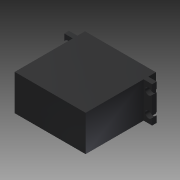
# Autodesk Inventor part: servo 33kg TGY-S8166M
Saved by Autodesk Inventor 2013 (Build 170138000, 138)
## iProperties
Created: 2013-03-06
Part Number: servo 33kg TGY-S8166M
Material: Generic
Document SubType Name: Modeling
Designer: Masta
Density: 1.41898 g/cm^3
Mass: 160 g
Surface Area: 160.569 cm^2
Volume: 112.757 cm^3
Author: Masta
Autodesk Inventor part; units mm, degrees
ref_plane "YZ Plane" through (0, 0, 0) normal (1, 0, 0) x (0, 1, 0)
ref_plane "XZ Plane" through (0, 0, 0) normal (0, 1, 0) x (-1, 0, 0)
ref_plane "XY Plane" through (0, 0, 0) normal (0, 0, 1) x (1, 0, 0)
sketch "Sketch1" plane through (0, 0, 0) normal (0, 1, 0) x (-1, 0, 0)
  line L0 (30.25, 15.25) -> (-30.25, 15.25)
  line L1 (-30.25, 15.25) -> (-30.25, -15.25)
  line L2 (-30.25, -15.25) -> (30.25, -15.25)
  line L3 (30.25, -15.25) -> (30.25, 15.25)
  line L4 (30.25, 15.25) -> (-30.25, -15.25) construction
  line L5 (-30.25, 15.25) -> (30.25, -15.25) construction
  line L6 (-37.5, 15.25) -> (-37.5, 9.75)
  line L7 (37.5, -15.25) -> (37.5, -9.75)
  line L8 (37.5, 15.25) -> (-37.5, -15.25) construction
  line L9 (-37.5, 15.25) -> (37.5, -15.25) construction
  line L10 (30.25, -15.25) -> (37.5, -15.25)
  line L11 (30.25, 15.25) -> (37.5, 15.25)
  line L12 (-30.25, 15.25) -> (-37.5, 15.25)
  line L13 (-30.25, -15.25) -> (-37.5, -15.25)
  line L14 (34.5, 8.5) -> (-34.5, 8.5) construction
  line L15 (-34.5, 8.5) -> (-34.5, -8.5) construction
  line L16 (-34.5, -8.5) -> (34.5, -8.5) construction
  line L17 (34.5, -8.5) -> (34.5, 8.5) construction
  line L18 (34.5, 8.5) -> (-34.5, -8.5) construction
  line L19 (-34.5, 8.5) -> (34.5, -8.5) construction
  circle A0 centre (-34.5, 8.5) radius 3
  line L20 (-37.5, 7.25) -> (-37.2272, 7.25)
  line L21 (-37.5, 9.75) -> (-37.2272, 9.75)
  line L22 (-30.25, 0) -> (30.25, 0) construction
  line L23 (0, 15.25) -> (0, -15.25) construction
  circle A1 centre (-34.5, -8.5) radius 3
  line L24 (-37.5, -7.25) -> (-37.2272, -7.25)
  line L25 (-37.5, -9.75) -> (-37.2272, -9.75)
  circle A2 centre (34.5, 8.5) radius 3
  line L26 (37.5, 7.25) -> (37.2272, 7.25)
  line L27 (37.5, 9.75) -> (37.2272, 9.75)
  line L28 (37.5, -9.75) -> (37.2272, -9.75)
  line L29 (37.5, -7.25) -> (37.2272, -7.25)
  circle A3 centre (34.5, -8.5) radius 3
  line L30 (-37.5, 7.25) -> (-37.5, -7.25)
  line L31 (-37.5, 9.75) -> (-37.5, 7.25)
  line L32 (-37.5, -9.75) -> (-37.5, -15.25)
  line L33 (-37.5, -7.25) -> (-37.5, -9.75)
  line L34 (37.5, -7.25) -> (37.5, 7.25)
  line L35 (37.5, -9.75) -> (37.5, -7.25)
  line L36 (37.5, 7.25) -> (37.5, 9.75)
  line L37 (37.5, 9.75) -> (37.5, 15.25)
  point P0 (0, 0)
  dimension "d0" = 60.5
  dimension "d1" = 30.5
  dimension "d2" = 75
  dimension "d3" = 69
  dimension "d4" = 17
  dimension "d12" = 2.5
  dimension "d13" = 6
  constraints: 76 end point, 32 parallel, 15 symmetric about line, 12 perpendicular, 10 midpoint, 8 point on circle, 4 centre point, 2 collinear, 2 horizontal, 1 coincident, 4 other
  measures "d0" distance of L2.end L1.end
  measures "d1" distance of L1.end L0.end
  measures "d2" distance of L7.start L8.end
  measures "d3" distance of L16.end L15.end
  measures "d4" distance of L15.end L14.end
  measures "d12" distance between parallel lines of L20 L21
  measures "d13" diameter of A0
extrude "Extrusion1" add sketch "Sketch1" along normal blind 10.5 and the other way blind 49.5 contours L3 L2 L1 L0
extrude "Extrusion2" add sketch "Sketch1" along normal blind 4 contours L11 L37 L27 A2 L26 L34 L29 A3 L28 L7 L10 L3 | L1 L13 L32 L25 A1 L24 L30 L20 A0 L21 L6 L12
sketch "Sketch2" plane through (0, 10.5, 0) normal (0, 1, 0) x (1, 0, 0)
  line L0 (-30.25, 15.25) -> (-30.25, -15.25) projected
  circle A0 centre (-15.25, 0) radius 7.5
  line L1 (-15.25, 0) -> (0, 0) construction
  dimension "d14" = 15
  dimension "d15" = 15
  constraints: 2 end point, 1 centre point, 1 perpendicular
  measures "d14" diameter of A0
  measures "d15" distance from line of L1.start L0
extrude "Extrusion3" add sketch "Sketch2" along normal blind 2
sketch "Sketch3" plane through (-15.25, 12.5, 0) normal (0, 1, 0) x (1, 0, 0)
  circle A0 centre (0, 0) radius 7.5 projected
  circle A1 centre (0, 0) radius 3.5
  point P0 (15.25, 0)
  dimension "d18" = 7
  constraints: 1 centre point, 1 coincident
  measures "d18" diameter of A1
extrude "Extrusion4" add sketch "Sketch3" along normal blind 6 contours A1
sketch "Sketch4" plane through (-30.25, -49.5, -15.25) normal (-1, 0, 0) x (0, 0, 1)
  line L0 (30.5, 49.5) -> (0, 49.5) projected
  line L1 (11.75, 25) -> (18.75, 25)
  line L2 (18.75, 25) -> (18.75, 29.5)
  line L3 (18.75, 29.5) -> (11.75, 29.5)
  line L4 (11.75, 29.5) -> (11.75, 25)
  line L5 (11.75, 25) -> (18.75, 29.5) construction
  line L6 (18.75, 25) -> (11.75, 29.5) construction
  line L7 (15.25, 49.5) -> (15.25, 27.25) construction
  dimension "d21" = 7
  dimension "d22" = 4.5
  dimension "d23" = 20
  constraints: 14 end point, 3 parallel, 2 midpoint, 1 horizontal, 1 perpendicular
  measures "d21" distance of L3.end L2.end
  measures "d22" distance of L2.end L1.end
  measures "d23" distance between parallel lines of L0 L3
extrude "Extrusion5" add sketch "Sketch4" along normal blind 7 draft -5
sketch "Sketch5" plane through (0, 0, 0) normal (0, 0, 1) x (1, 0, 0)
  line L0 (37.5, 4) -> (37.5, 0) projected
  line L1 (37.5, 0) -> (30.25, 0) projected
  line L2 (30.25, 0) -> (30.25, -49.5) projected
  line L3 (30.25, -49.5) -> (-30.25, -49.5) projected
  line L4 (-30.25, -24.5) -> (-37.25, -23.8876) projected
  line L5 (-37.25, -23.8876) -> (-37.25, -20.6124) projected
  line L6 (-37.25, -20.6124) -> (-30.25, -20) projected
  line L7 (-30.25, -20) -> (-30.25, 0) projected
  line L8 (-30.25, 0) -> (-37.5, 0) projected
  line L9 (-37.5, 0) -> (-37.5, 4) projected
  line L10 (-37.5, 4) -> (-30.25, 4) projected
  line L11 (-30.25, 4) -> (-30.25, 10.5) projected
  line L12 (-30.25, 10.5) -> (-22.75, 10.5) projected
  line L13 (-22.75, 10.5) -> (-22.75, 12.5) projected
  line L14 (-22.75, 12.5) -> (-18.75, 12.5) projected
  line L15 (-18.75, 12.5) -> (-18.75, 18.5) projected
  line L16 (-18.75, 18.5) -> (-11.75, 18.5) projected
  line L17 (-11.75, 18.5) -> (-11.75, 12.5) projected
  line L18 (-11.75, 12.5) -> (-7.75, 12.5) projected
  line L19 (-7.75, 12.5) -> (-7.75, 10.5) projected
  line L20 (-7.75, 10.5) -> (30.25, 10.5) projected
  line L21 (30.25, 10.5) -> (30.25, 4) projected
  line L22 (30.25, 4) -> (37.5, 4) projected
  line L23 (-37.5, 4) -> (-30.25, 5.1)
  line L24 (30.25, 5.1) -> (37.5, 4)
  line L25 (-30.25, -49.5) -> (-30.25, -24.5) projected
  point P0 (0, 0)
  point P1 (-20.25, -27)
  dimension "d26" = 1.1
  constraints: 4 end point, 2 point on line, 1 equal length
  measures "d26" distance of L23.end L10.end
extrude "Extrusion6" add sketch "Sketch5" along normal mid plane 1.3 contours L22 L21 L24 | L23 L11 L10
sketch "Sketch6" plane through (0, 10.5, 0) normal (0, 1, 0) x (1, 0, 0)
  line L0 (12.3297, -9.4801) -> (12.3297, 4.6475) construction
  line L1 (12.3297, 4.6475) -> (15.9034, 4.6475) construction
  line L2 (15.9034, 4.6475) -> (15.9034, -9.4801) construction
  line L3 (15.9034, -9.4801) -> (12.3297, -9.4801) construction
  line L4 (14.8586, -8.6525) -> (12.6784, -8.6525)
  line L5 (12.6784, -8.6525) -> (12.6784, -9.4821)
  line L6 (12.6784, -9.4821) -> (12.3858, -9.4821)
  line L7 (12.3858, -9.4821) -> (12.3858, -7.4942)
  line L8 (12.3858, -7.4942) -> (12.6784, -7.4942)
  line L9 (12.6784, -7.4942) -> (12.6784, -8.3238)
  line L10 (12.6784, -8.3238) -> (14.8586, -8.3238)
  line L11 (14.8586, -8.3238) -> (14.8586, -8.6525)
  spline S0 degree 2 poles (14.9067, -6.2077) (14.9067, -6.4702) (14.7464, -6.9051) (14.5841, -7.0614) knots 0 0 0 1 2 2 2
  spline S1 degree 2 poles (14.5841, -7.0614) (14.4198, -7.2177) (13.9348, -7.384) (13.6202, -7.384) knots 0 0 0 1 2 2 2
  spline S2 degree 2 poles (13.6202, -7.384) (13.3216, -7.384) (12.8487, -7.2157) (12.6804, -7.0594) knots 0 0 0 1 2 2 2
  spline S3 degree 2 poles (12.6804, -7.0594) (12.5181, -6.9091) (12.3417, -6.4682) (12.3417, -6.2057) knots 0 0 0 1 2 2 2
  spline S4 degree 2 poles (12.3417, -6.2057) (12.3417, -6.0795) (12.3778, -5.851) (12.4098, -5.7468) knots 0 0 0 1 2 2 2
  spline S5 degree 2 poles (12.4098, -5.7468) (12.4339, -5.6627) (12.5221, -5.4583) (12.5541, -5.3961) knots 0 0 0 1 2 2 2
  line L12 (12.5541, -5.3961) -> (12.9509, -5.3961)
  line L13 (12.9509, -5.3961) -> (12.9509, -5.4242)
  spline S6 degree 2 poles (12.9509, -5.4242) (12.8968, -5.4863) (12.7986, -5.6166) (12.7425, -5.7368) knots 0 0 0 1 2 2 2
  spline S7 degree 2 poles (12.7425, -5.7368) (12.6924, -5.837) (12.6263, -6.0955) (12.6263, -6.2438) knots 0 0 0 1 2 2 2
  spline S8 degree 2 poles (12.6263, -6.2438) (12.6263, -6.6005) (13.1633, -7.0413) (13.6102, -7.0413) knots 0 0 0 1 2 2 2
  spline S9 degree 2 poles (13.6102, -7.0413) (13.8587, -7.0413) (14.2314, -6.9251) (14.3596, -6.8149) knots 0 0 0 1 2 2 2
  spline S10 degree 2 poles (14.3596, -6.8149) (14.4879, -6.7087) (14.6222, -6.4081) (14.6222, -6.2197) knots 0 0 0 1 2 2 2
  spline S11 degree 2 poles (14.6222, -6.2197) (14.6222, -6.0815) (14.5821, -5.8049) (14.542, -5.7107) knots 0 0 0 1 2 2 2
  line L14 (14.542, -5.7107) -> (13.9028, -5.7107)
  line L15 (13.9028, -5.7107) -> (13.9028, -6.2839)
  line L16 (13.9028, -6.2839) -> (13.6142, -6.2839)
  line L17 (13.6142, -6.2839) -> (13.6142, -5.3861)
  line L18 (13.6142, -5.3861) -> (14.6943, -5.3861)
  spline S12 degree 2 poles (14.6943, -5.3861) (14.7224, -5.4482) (14.8085, -5.6607) (14.8346, -5.7508) knots 0 0 0 1 2 2 2
  spline S13 degree 2 poles (14.8346, -5.7508) (14.8706, -5.8731) (14.9067, -6.0694) (14.9067, -6.2077) knots 0 0 0 1 2 2 2
  line L19 (12.3858, -3.2419) -> (13.7645, -4.0776)
  line L20 (13.7645, -4.0776) -> (14.8586, -4.0776)
  line L21 (14.8586, -4.0776) -> (14.8586, -4.4062)
  line L22 (14.8586, -4.4062) -> (13.7985, -4.4062)
  line L23 (13.7985, -4.4062) -> (12.3858, -5.2418)
  line L24 (12.3858, -5.2418) -> (12.3858, -4.8771)
  line L25 (12.3858, -4.8771) -> (13.4739, -4.2399)
  line L26 (13.4739, -4.2399) -> (12.3858, -3.5906)
  line L27 (12.3858, -3.5906) -> (12.3858, -3.2419)
  line L28 (13.9268, -2.1779) -> (13.9268, -3.1137)
  line L29 (13.9268, -3.1137) -> (13.6262, -3.1137)
  line L30 (13.6262, -3.1137) -> (13.6262, -2.1779)
  line L31 (13.6262, -2.1779) -> (13.9268, -2.1779)
  spline S14 degree 2 poles (14.9027, -1.0897) (14.9027, -1.3583) (14.7905, -1.735) (14.7103, -1.9013) knots 0 0 0 1 2 2 2
  line L32 (14.7103, -1.9013) -> (14.2975, -1.9013)
  line L33 (14.2975, -1.9013) -> (14.2975, -1.8773)
  spline S15 degree 2 poles (14.2975, -1.8773) (14.4498, -1.715) (14.6181, -1.3041) (14.6181, -1.1138) knots 0 0 0 1 2 2 2
  spline S16 degree 2 poles (14.6181, -1.1138) (14.6181, -0.8412) (14.3917, -0.5627) (14.2053, -0.5627) knots 0 0 0 1 2 2 2
  spline S17 degree 2 poles (14.2053, -0.5627) (14.0571, -0.5627) (13.8727, -0.709) (13.8266, -0.8673) knots 0 0 0 1 2 2 2
  spline S18 degree 2 poles (13.8266, -0.8673) (13.7945, -0.9815) (13.7505, -1.1719) (13.7144, -1.3142) knots 0 0 0 1 2 2 2
  spline S19 degree 2 poles (13.7144, -1.3142) (13.6803, -1.4424) (13.5781, -1.6448) (13.496, -1.723) knots 0 0 0 1 2 2 2
  spline S20 degree 2 poles (13.496, -1.723) (13.4138, -1.7991) (13.1934, -1.8833) (13.0491, -1.8833) knots 0 0 0 1 2 2 2
  spline S21 degree 2 poles (13.0491, -1.8833) (12.7485, -1.8833) (12.3417, -1.4144) (12.3417, -1.0517) knots 0 0 0 1 2 2 2
  spline S22 degree 2 poles (12.3417, -1.0517) (12.3417, -0.8433) (12.4239, -0.4745) (12.502, -0.3162) knots 0 0 0 1 2 2 2
  line L34 (12.502, -0.3162) -> (12.8948, -0.3162)
  line L35 (12.8948, -0.3162) -> (12.8948, -0.3403)
  spline S23 degree 2 poles (12.8948, -0.3403) (12.7866, -0.4585) (12.6263, -0.8272) (12.6263, -1.0296) knots 0 0 0 1 2 2 2
  spline S24 degree 2 poles (12.6263, -1.0296) (12.6263, -1.2581) (12.8407, -1.5406) (13.015, -1.5406) knots 0 0 0 1 2 2 2
  spline S25 degree 2 poles (13.015, -1.5406) (13.1713, -1.5406) (13.3577, -1.3743) (13.3998, -1.218) knots 0 0 0 1 2 2 2
  spline S26 degree 2 poles (13.3998, -1.218) (13.4278, -1.1138) (13.5, -0.8112) (13.53, -0.711) knots 0 0 0 1 2 2 2
  spline S27 degree 2 poles (13.53, -0.711) (13.6082, -0.4565) (13.9228, -0.22) (14.1532, -0.22) knots 0 0 0 1 2 2 2
  spline S28 degree 2 poles (14.1532, -0.22) (14.2995, -0.22) (14.5801, -0.3383) (14.6783, -0.4445) knots 0 0 0 1 2 2 2
  spline S29 degree 2 poles (14.6783, -0.4445) (14.7865, -0.5627) (14.9027, -0.8633) (14.9027, -1.0897) knots 0 0 0 1 2 2 2
  spline S30 degree 2 poles (14.9147, 0.7919) (14.9147, 0.6076) (14.8045, 0.305) (14.7023, 0.1988) knots 0 0 0 1 2 2 2
  spline S31 degree 2 poles (14.7023, 0.1988) (14.6021, 0.0946) (14.3296, -0.0136) (14.1753, -0.0136) knots 0 0 0 1 2 2 2
  spline S32 degree 2 poles (14.1753, -0.0136) (13.9749, -0.0136) (13.6382, 0.2008) (13.538, 0.4052) knots 0 0 0 1 2 2 2
  line L36 (13.538, 0.4052) -> (13.528, 0.4052)
  spline S33 degree 2 poles (13.528, 0.4052) (13.4218, 0.2228) (13.1693, 0.0465) (12.981, 0.0465) knots 0 0 0 1 2 2 2
  spline S34 degree 2 poles (12.981, 0.0465) (12.7024, 0.0465) (12.3297, 0.4673) (12.3297, 0.7919) knots 0 0 0 1 2 2 2
  spline S35 degree 2 poles (12.3297, 0.7919) (12.3297, 1.1286) (12.6824, 1.5354) (12.9589, 1.5354) knots 0 0 0 1 2 2 2
  spline S36 degree 2 poles (12.9589, 1.5354) (13.1252, 1.5354) (13.4499, 1.341) (13.542, 1.1587) knots 0 0 0 1 2 2 2
  line L37 (13.542, 1.1587) -> (13.5521, 1.1587)
  spline S37 degree 2 poles (13.5521, 1.1587) (13.6523, 1.3751) (13.9408, 1.5975) (14.1693, 1.5975) knots 0 0 0 1 2 2 2
  spline S38 degree 2 poles (14.1693, 1.5975) (14.4859, 1.5975) (14.9147, 1.1366) (14.9147, 0.7919) knots 0 0 0 1 2 2 2
  spline S39 degree 2 poles (14.2013, 1.2568) (14.049, 1.2568) (13.8687, 1.1366) (13.7765, 0.9663) knots 0 0 0 1 2 2 2
  spline S40 degree 2 poles (13.7765, 0.9663) (13.7444, 0.9102) (13.6703, 0.7218) (13.6222, 0.6036) knots 0 0 0 1 2 2 2
  spline S41 degree 2 poles (13.6222, 0.6036) (13.7124, 0.4673) (13.9809, 0.321) (14.1512, 0.321) knots 0 0 0 1 2 2 2
  spline S42 degree 2 poles (14.1512, 0.321) (14.3757, 0.321) (14.6682, 0.5916) (14.6682, 0.7959) knots 0 0 0 1 2 2 2
  spline S43 degree 2 poles (14.6682, 0.7959) (14.6682, 1.0044) (14.4178, 1.2568) (14.2013, 1.2568) knots 0 0 0 1 2 2 2
  spline S44 degree 2 poles (12.9629, 1.2108) (12.7966, 1.2108) (12.5742, 0.9883) (12.5742, 0.7899) knots 0 0 0 1 2 2 2
  spline S45 degree 2 poles (12.5742, 0.7899) (12.5742, 0.6096) (12.7725, 0.3791) (12.9429, 0.3791) knots 0 0 0 1 2 2 2
  spline S46 degree 2 poles (12.9429, 0.3791) (13.0651, 0.3791) (13.2355, 0.4974) (13.3036, 0.6156) knots 0 0 0 1 2 2 2
  spline S47 degree 2 poles (13.3036, 0.6156) (13.3316, 0.6657) (13.4298, 0.8781) (13.4579, 0.9643) knots 0 0 0 1 2 2 2
  spline S48 degree 2 poles (13.4579, 0.9643) (13.3477, 1.1086) (13.1132, 1.2108) (12.9629, 1.2108) knots 0 0 0 1 2 2 2
  line L38 (14.8586, 3.3008) -> (14.8586, 2.0945)
  line L39 (14.8586, 2.0945) -> (14.6061, 2.0945)
  line L40 (14.6061, 2.0945) -> (14.6061, 2.5434)
  line L41 (14.6061, 2.5434) -> (12.9489, 2.5434)
  line L42 (12.9489, 2.5434) -> (12.9489, 2.0945)
  line L43 (12.9489, 2.0945) -> (12.7224, 2.0945)
  spline S49 degree 2 poles (12.7224, 2.0945) (12.7224, 2.349) (12.5782, 2.5894) (12.3778, 2.6055) knots 0 0 0 1 2 2 2
  line L44 (12.3778, 2.6055) -> (12.3778, 2.862)
  line L45 (12.3778, 2.862) -> (14.6061, 2.862)
  line L46 (14.6061, 2.862) -> (14.6061, 3.3008)
  line L47 (14.6061, 3.3008) -> (14.8586, 3.3008)
  spline S50 degree 2 poles (14.0571, 5.3188) (14.2474, 5.3188) (14.5701, 5.1925) (14.6783, 5.0863) knots 0 0 0 1 2 2 2
  spline S51 degree 2 poles (14.6783, 5.0863) (14.7925, 4.9761) (14.9107, 4.6996) (14.9107, 4.5332) knots 0 0 0 1 2 2 2
  spline S52 degree 2 poles (14.9107, 4.5332) (14.9107, 4.3669) (14.7985, 4.0924) (14.6863, 3.9882) knots 0 0 0 1 2 2 2
  spline S53 degree 2 poles (14.6863, 3.9882) (14.552, 3.8599) (14.1011, 3.7156) (13.7725, 3.7156) knots 0 0 0 1 2 2 2
  spline S54 degree 2 poles (13.7725, 3.7156) (13.4499, 3.7156) (12.9309, 3.8479) (12.7385, 3.9862) knots 0 0 0 1 2 2 2
  spline S55 degree 2 poles (12.7385, 3.9862) (12.5501, 4.1204) (12.3397, 4.5453) (12.3397, 4.8238) knots 0 0 0 1 2 2 2
  spline S56 degree 2 poles (12.3397, 4.8238) (12.3397, 4.906) (12.3557, 5.0503) (12.3738, 5.1044) knots 0 0 0 1 2 2 2
  line L48 (12.3738, 5.1044) -> (12.6924, 5.1044)
  line L49 (12.6924, 5.1044) -> (12.6924, 5.0903)
  spline S57 degree 2 poles (12.6924, 5.0903) (12.6683, 5.0442) (12.6263, 4.8759) (12.6263, 4.7797) knots 0 0 0 1 2 2 2
  spline S58 degree 2 poles (12.6263, 4.7797) (12.6263, 4.4711) (13.0431, 4.0924) (13.4519, 4.0563) knots 0 0 0 1 2 2 2
  spline S59 degree 2 poles (13.4519, 4.0563) (13.3697, 4.1745) (13.2795, 4.423) (13.2795, 4.5713) knots 0 0 0 1 2 2 2
  spline S60 degree 2 poles (13.2795, 4.5713) (13.2795, 4.7156) (13.3376, 4.932) (13.4258, 5.0503) knots 0 0 0 1 2 2 2
  spline S61 degree 2 poles (13.4258, 5.0503) (13.528, 5.1865) (13.8446, 5.3188) (14.0571, 5.3188) knots 0 0 0 1 2 2 2
  spline S62 degree 2 poles (14.0711, 4.9821) (13.9188, 4.9821) (13.7124, 4.902) (13.6402, 4.8138) knots 0 0 0 1 2 2 2
  spline S63 degree 2 poles (13.6402, 4.8138) (13.5881, 4.7477) (13.5541, 4.5833) (13.5541, 4.4972) knots 0 0 0 1 2 2 2
  spline S64 degree 2 poles (13.5541, 4.4972) (13.5541, 4.3809) (13.6242, 4.1625) (13.6903, 4.0563) knots 0 0 0 1 2 2 2
  spline S65 degree 2 poles (13.6903, 4.0563) (13.7264, 4.0543) (13.7945, 4.0503) (13.8466, 4.0503) knots 0 0 0 1 2 2 2
  spline S66 degree 2 poles (13.8466, 4.0503) (14.1031, 4.0503) (14.4178, 4.1505) (14.4999, 4.2266) knots 0 0 0 1 2 2 2
  spline S67 degree 2 poles (14.4999, 4.2266) (14.5781, 4.2968) (14.6402, 4.4491) (14.6402, 4.5352) knots 0 0 0 1 2 2 2
  spline S68 degree 2 poles (14.6402, 4.5352) (14.6402, 4.7356) (14.3556, 4.9821) (14.0711, 4.9821) knots 0 0 0 1 2 2 2
  spline S69 degree 2 poles (14.0571, 7.1744) (14.2474, 7.1744) (14.5701, 7.0482) (14.6783, 6.9419) knots 0 0 0 1 2 2 2
  spline S70 degree 2 poles (14.6783, 6.9419) (14.7925, 6.8317) (14.9107, 6.5552) (14.9107, 6.3889) knots 0 0 0 1 2 2 2
  spline S71 degree 2 poles (14.9107, 6.3889) (14.9107, 6.2225) (14.7985, 5.948) (14.6863, 5.8438) knots 0 0 0 1 2 2 2
  spline S72 degree 2 poles (14.6863, 5.8438) (14.552, 5.7156) (14.1011, 5.5713) (13.7725, 5.5713) knots 0 0 0 1 2 2 2
  spline S73 degree 2 poles (13.7725, 5.5713) (13.4499, 5.5713) (12.9309, 5.7035) (12.7385, 5.8418) knots 0 0 0 1 2 2 2
  spline S74 degree 2 poles (12.7385, 5.8418) (12.5501, 5.9761) (12.3397, 6.4009) (12.3397, 6.6794) knots 0 0 0 1 2 2 2
  spline S75 degree 2 poles (12.3397, 6.6794) (12.3397, 6.7616) (12.3557, 6.9059) (12.3738, 6.96) knots 0 0 0 1 2 2 2
  line L50 (12.3738, 6.96) -> (12.6924, 6.96)
  line L51 (12.6924, 6.96) -> (12.6924, 6.946)
  spline S76 degree 2 poles (12.6924, 6.946) (12.6683, 6.8999) (12.6263, 6.7315) (12.6263, 6.6353) knots 0 0 0 1 2 2 2
  spline S77 degree 2 poles (12.6263, 6.6353) (12.6263, 6.3267) (13.0431, 5.948) (13.4519, 5.9119) knots 0 0 0 1 2 2 2
  spline S78 degree 2 poles (13.4519, 5.9119) (13.3697, 6.0302) (13.2795, 6.2786) (13.2795, 6.4269) knots 0 0 0 1 2 2 2
  spline S79 degree 2 poles (13.2795, 6.4269) (13.2795, 6.5712) (13.3376, 6.7876) (13.4258, 6.9059) knots 0 0 0 1 2 2 2
  spline S80 degree 2 poles (13.4258, 6.9059) (13.528, 7.0421) (13.8446, 7.1744) (14.0571, 7.1744) knots 0 0 0 1 2 2 2
  spline S81 degree 2 poles (14.0711, 6.8377) (13.9188, 6.8377) (13.7124, 6.7576) (13.6402, 6.6694) knots 0 0 0 1 2 2 2
  spline S82 degree 2 poles (13.6402, 6.6694) (13.5881, 6.6033) (13.5541, 6.439) (13.5541, 6.3528) knots 0 0 0 1 2 2 2
  spline S83 degree 2 poles (13.5541, 6.3528) (13.5541, 6.2366) (13.6242, 6.0181) (13.6903, 5.9119) knots 0 0 0 1 2 2 2
  spline S84 degree 2 poles (13.6903, 5.9119) (13.7264, 5.9099) (13.7945, 5.9059) (13.8466, 5.9059) knots 0 0 0 1 2 2 2
  spline S85 degree 2 poles (13.8466, 5.9059) (14.1031, 5.9059) (14.4178, 6.0061) (14.4999, 6.0823) knots 0 0 0 1 2 2 2
  spline S86 degree 2 poles (14.4999, 6.0823) (14.5781, 6.1524) (14.6402, 6.3047) (14.6402, 6.3909) knots 0 0 0 1 2 2 2
  spline S87 degree 2 poles (14.6402, 6.3909) (14.6402, 6.5913) (14.3556, 6.8377) (14.0711, 6.8377) knots 0 0 0 1 2 2 2
  line L52 (14.8586, 9.6572) -> (14.8586, 9.3286)
  line L53 (14.8586, 9.3286) -> (12.7285, 9.3286)
  line L54 (12.7285, 9.3286) -> (14.1773, 8.6833)
  line L55 (14.1773, 8.6833) -> (14.1773, 8.483)
  line L56 (14.1773, 8.483) -> (12.7285, 7.8437)
  line L57 (12.7285, 7.8437) -> (14.8586, 7.8437)
  line L58 (14.8586, 7.8437) -> (14.8586, 7.5371)
  line L59 (14.8586, 7.5371) -> (12.3858, 7.5371)
  line L60 (12.3858, 7.5371) -> (12.3858, 7.986)
  line L61 (12.3858, 7.986) -> (13.7625, 8.6032)
  line L62 (13.7625, 8.6032) -> (12.3858, 9.2004)
  line L63 (12.3858, 9.2004) -> (12.3858, 9.6572)
  line L64 (12.3858, 9.6572) -> (14.8586, 9.6572)
  point P0 (0, 0)
  constraints: 2 other
emboss "Emboss1" sketch "Sketch6" operation cut depth 0.1 direction (0, -1, 0)
hole "Hole1" at (-15.25, 18.5, 0) direction (0, -1, 0) diameter 2.459 depth 8 tip angle 118 thread size "M3x0.5" class "6H" standard "ISO Metric profile"
body "Solid1"
